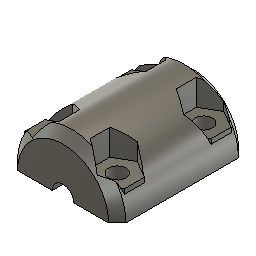
Z_coupler_new_8mm_v3 (Autodesk Fusion 360 design; units mm, degrees)
Autodesk Fusion 360 part; units mm, degrees
note: some values were not read from the file. Set by a fixed rule: which sketch regions a step uses.
sketch "Sketch1" plane through (0, 0, 0) normal (0, 0, 1) x (1, 0, 0)
  circle A0 centre (0, 0) radius 2.5
  circle A1 centre (0, 0) radius 12.5
  circle A2 centre (0, 0) radius 4
  line L0 (-12.5, 0) -> (12.5, 0)
  dimension "d1" = 5
  dimension "d2" = 25
  dimension "d3" = 8
  measures "d1" diameter of A0
  measures "d2" diameter of A1
  measures "d3" diameter of A2
extrude "Extrude1" add sketch "Sketch1" along normal blind 15 contours A0 A2 L0 | A1 A2 L0 picked at (-3.4758, 0.3229) picked at (-7.4744, 6.0881)
extrude "Extrude2" add sketch "Sketch1" against normal blind 15 contours A1 A2 L0 picked at (-7.4744, 6.0881)
sketch "Sketch2" plane through (0, 0, 0) normal (0, -1, 0) x (1, 0, 0)
  line L0 (-4, 0) -> (-2.5, 0)
  line L1 (-2.5, 0) -> (-2.5, 15)
  line L2 (-2.5, 15) -> (-12.5, 15)
  line L3 (-12.5, 15) -> (-12.5, -15)
  line L4 (-12.5, -15) -> (-4, -15)
  line L5 (-4, -15) -> (-4, 0)
  circle A0 centre (-7.5, 10) radius 2
  circle A1 centre (7.5, 10) radius 2
  line L6 (2.5, 15) -> (12.5, 15)
  line L7 (12.5, -15) -> (12.5, 15)
  circle A2 centre (-7.5, -10) radius 2
  circle A3 centre (7.5, -10) radius 2
  line L8 (12.5, -15) -> (4, -15)
  line L9 (-3.5, 7.6906) -> (-3.5, 12.3094)
  line L10 (-3.5, 12.3094) -> (-7.5, 14.6188)
  line L11 (-7.5, 14.6188) -> (-11.5, 12.3094)
  line L12 (-11.5, 12.3094) -> (-11.5, 7.6906)
  line L13 (-11.5, 7.6906) -> (-7.5, 5.3812)
  line L14 (-7.5, 5.3812) -> (-3.5, 7.6906)
  line L15 (11.5, 7.6906) -> (11.5, 12.3094)
  line L16 (11.5, 12.3094) -> (7.5, 14.6188)
  line L17 (7.5, 14.6188) -> (3.5, 12.3094)
  line L18 (3.5, 12.3094) -> (3.5, 7.6906)
  line L19 (3.5, 7.6906) -> (7.5, 5.3812)
  line L20 (7.5, 5.3812) -> (11.5, 7.6906)
  line L21 (-3.5, -12.3094) -> (-3.5, -7.6906)
  line L22 (-3.5, -7.6906) -> (-7.5, -5.3812)
  line L23 (-7.5, -5.3812) -> (-11.5, -7.6906)
  line L24 (-11.5, -7.6906) -> (-11.5, -12.3094)
  line L25 (-11.5, -12.3094) -> (-7.5, -14.6188)
  line L26 (-7.5, -14.6188) -> (-3.5, -12.3094)
  line L27 (11.5, -12.3094) -> (11.5, -7.6906)
  line L28 (11.5, -7.6906) -> (7.5, -5.3812)
  line L29 (7.5, -5.3812) -> (3.5, -7.6906)
  line L30 (3.5, -7.6906) -> (3.5, -12.3094)
  line L31 (3.5, -12.3094) -> (7.5, -14.6188)
  line L32 (7.5, -14.6188) -> (11.5, -12.3094)
  dimension "d8" = 4
  dimension "d9" = 4
  dimension "d10" = 5
  dimension "d11" = 5
  dimension "d12" = 5
  dimension "d13" = 5
  dimension "d14" = 4
  dimension "d15" = 4
  dimension "d16" = 5
  dimension "d17" = 5
  dimension "d18" = 5
  dimension "d19" = 5
  dimension "d20" = 4
  dimension "d21" = 4
  dimension "d22" = 4
  dimension "d23" = 4
  measures "d8" diameter of A0
  measures "d9" diameter of A1
  measures "d10" distance of L2
  measures "d11" distance of L6
  measures "d12" distance of L7
  measures "d13" distance of L3
  measures "d14" diameter of A2
  measures "d15" diameter of A3
  measures "d16" distance of L8
  measures "d17" distance of L4
  measures "d18" distance of L3
  measures "d19" distance of L7
  measures "d20" distance of L14
  measures "d21" distance of L20
  measures "d22" distance of L26
  measures "d23" distance of L32
extrude "Extrude3" cut sketch "Sketch2" against normal blind 18 contours L5 L21 L22 L26 | L5 L22 L23 L24 L25 L26 | A0 | A1 | A2 | A3 | L9 L10 L11 L12 L13 L14 | L15 L16 L17 L18 L19 L20 | L27 L28 L29 L30 L31 L32
extrude "Extrude4" add sketch "Sketch2" against normal blind 6 contours L5 L21 L22 L26 | L5 L22 L23 L24 L25 L26 | L9 L10 L11 L12 L13 L14 | L15 L16 L17 L18 L19 L20 | L27 L28 L29 L30 L31 L32
extrude "Extrude5" cut sketch "Sketch1" against normal blind 33 contours A0 A2 L0 picked at (-3.4758, 0.3229)
chamfer "Chamfer1" distance 2 angle 45 2 edges at (0, 12.5, 15) (0, 12.5, -15)
